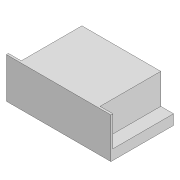
# Autodesk Inventor part: POWER SUPPLY
Saved by Autodesk Inventor 2020 (Build 240168000, 168)
## iProperties
Created: 2020-04-09
Part Number: POWER SUPPLY
Material: Generic
Document SubType Name: Modeling
Designer: angusaitken
Density: 1 g/cm^3
Appearance: Default
Description: RPS-120-12
Author: angusaitken
Autodesk Inventor part; units mm, degrees
ref_plane "YZ Plane" through (0, 0, 0) normal (1, 0, 0) x (0, 1, 0)
ref_plane "XZ Plane" through (0, 0, 0) normal (0, 1, 0) x (-1, 0, 0)
ref_plane "XY Plane" through (0, 0, 0) normal (0, 0, 1) x (1, 0, 0)
sketch "Sketch1" plane through (0, 0, 0) normal (0, 1, 0) x (-1, 0, 0)
  line L0 (0, 0) -> (103.4, 0)
  line L1 (103.4, 0) -> (103.4, -62)
  line L2 (103.4, -62) -> (0, -62)
  line L3 (0, -62) -> (0, 0)
  dimension "d0" = 103.4
  dimension "d1" = 62
  constraints: 8 end point, 2 parallel, 1 horizontal, 1 perpendicular
  measures "d0" distance of L1.end L2.end
  measures "d1" distance of L0.end L1.end
extrude "Extrusion1" add sketch "Sketch1" along normal blind 40
sketch "Sketch2" plane through (0, 0, -62) normal (0, 0, -1) x (-1, 0, 0)
  line L0 (103.4, 40) -> (0, 40) projected
  line L1 (51.7, 40) -> (90.7, 40)
  line L2 (103.4, 0) -> (103.4, 40) projected
  line L3 (90.7, 40) -> (103.4, 40)
  line L4 (103.4, 40) -> (103.4, 10.0001)
  line L5 (103.4, 10.0001) -> (90.7, 10.0001)
  line L6 (90.7, 10.0001) -> (90.7, 40)
  line L7 (51.7, 40) -> (51.7, 19.0962)
  line L8 (0, 10.0001) -> (12.7, 10.0001)
  line L9 (12.7, 10.0001) -> (12.7, 40)
  line L10 (0, 40) -> (103.4, 40)
  line L11 (0, 0) -> (0, 40)
  dimension "d4" = 39
  constraints: 20 end point, 6 symmetric about line, 2 parallel, 2 point on line, 1 horizontal, 1 midpoint, 1 perpendicular, 1 vertical
  measures "d4" distance of L1.start L1.end
extrude "Extrusion2" cut sketch "Sketch2" against normal blind 60
body "Solid1"
